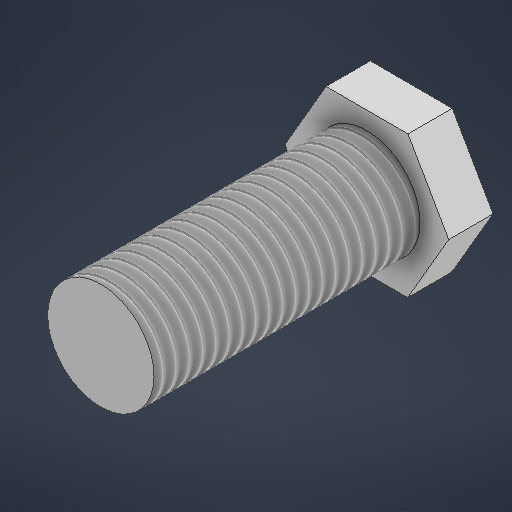
# Autodesk Inventor part: Part10
Saved by Autodesk Inventor 2026 (Build 300175000, 175)
## iProperties
Created: 2025-05-08
Part Number: Part10
Material: Generic
Document SubType Name: Modeling
Designer: Ritul Kumari
Density: 1 g/cm^3
Appearance: Default
Author: Ritul Kumari
Autodesk Inventor part; units mm, degrees
ref_plane "YZ Plane" through (0, 0, 0) normal (1, 0, 0) x (0, 1, 0)
ref_plane "XZ Plane" through (0, 0, 0) normal (0, 1, 0) x (-1, 0, 0)
ref_plane "XY Plane" through (0, 0, 0) normal (0, 0, 1) x (1, 0, 0)
sketch "Sketch1" plane through (0, 0, 0) normal (0, 0, 1) x (1, 0, 0)
  line L0 (4.5991, -8.0114) -> (-4.6385, -7.9886)
  line L1 (-4.6385, -7.9886) -> (-9.2376, 0.0227)
  line L2 (-9.2376, 0.0227) -> (-4.5991, 8.0114)
  line L3 (-4.5991, 8.0114) -> (4.6385, 7.9886)
  line L4 (4.6385, 7.9886) -> (9.2376, -0.0227)
  line L5 (9.2376, -0.0227) -> (4.5991, -8.0114)
  point P0 (0, 0)
  point P1 (0, 0)
  point P2 (-0.0197, -8)
  point P3 (0.0197, 8)
  dimension "d0" = 16
  constraints: 12 end point, 2 midpoint, 1 coincident, 13 other
  measures "d0" vertical distance of point (-0.02, -8) point (0.02, 8)
extrude "Extrusion1" add sketch "Sketch1" along normal blind 5
sketch "Sketch2" plane through (0, 0, 5) normal (0, 0, 1) x (1, 0, 0)
  circle A0 centre (0, 0) radius 6
  dimension "d3" = 12
  constraints: 1 centre point, 1 coincident
  measures "d3" diameter of A0
extrude "Extrusion2" add sketch "Sketch2" along normal blind 30
thread "Thread1" size "M12x1.5" class "6g" standard "ANSI Metric M Profile" full length
thread "Thread2" size "M12x1.5" class "6g" standard "ANSI Metric M Profile" full length
body "Solid1"
